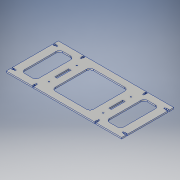
# Autodesk Inventor part: Hopper Bottom Brace
Saved by Autodesk Inventor 2018 (Build 220112000, 112)
## iProperties
Created: 2013-10-08
Part Number: Hopper Bottom Brace
Material: Aluminum 6061
Document SubType Name: Modeling
Designer: Gabriel Smolnycki
Mass: 299.366 g
Surface Area: 651.04 cm^2
Volume: 110.876 cm^3
Density: 2.7 g/cm^3
Appearance: Aluminum - Flat
Sending System: SolidWorks 2017
Last Author: Gabriel Smolnycki
Last Saved: 2017-09-14
Author: Gabriel Smolnycki
Autodesk Inventor part; units mm, degrees
ref_plane "YZ Plane" through (0, 0, 0) normal (1, 0, 0) x (0, 1, 0)
ref_plane "XY Plane" through (0, 0, 0) normal (0, 0, 1) x (1, 0, 0)
ref_plane "Work Plane1" through (0, -4, 0) normal (0, 1, 0) x (-1, 0, 0)
sketch "Sketch1" plane through (0, -4, 0) normal (0, 1, 0) x (-1, 0, 0)
  line L0 (-91.75, 75) -> (-91.75, 72)
  line L1 (88.25, 63) -> (91.75, 63)
  line L2 (163, 57.25) -> (163, 58.25)
  line L3 (91.75, -72) -> (92.75, -72)
  line L4 (-91.75, -63) -> (-91.75, -68)
  line L5 (-163, -58.25) -> (-166, -58.25)
  line L6 (143, -55) -> (143, 55)
  line L7 (-163, 61.75) -> (-166, 61.75)
  line L8 (87.25, 72) -> (87.25, 68)
  line L9 (154, 58.25) -> (159, 58.25)
  line L10 (166, -75) -> (166, -61.75)
  line L11 (-87.25, -68) -> (-88.25, -68)
  line L12 (-159, -58.25) -> (-159, -57.25)
  line L13 (81.5, -20) -> (81.5, 20)
  line L14 (-74.5, 20) -> (-81.5, 20)
  line L15 (-159, 61.75) -> (-159, 62.75)
  line L16 (88.25, 75) -> (-88.25, 75)
  line L17 (159, 62.75) -> (159, 61.75)
  line L18 (159, -62.75) -> (163, -62.75)
  line L19 (-88.25, -75) -> (-88.25, -72)
  line L20 (-159, -61.75) -> (-154, -61.75)
  line L21 (55, -55) -> (55, 55)
  line L22 (-159, 58.25) -> (-154, 58.25)
  line L23 (-87.25, 68) -> (-87.25, 72)
  line L24 (166, 61.75) -> (163, 61.75)
  line L25 (154, -58.25) -> (154, -61.75)
  line L26 (87.25, -72) -> (88.25, -72)
  line L27 (-163, -61.75) -> (-163, -62.75)
  line L28 (-163, 58.25) -> (-163, 57.25)
  line L29 (-91.75, 63) -> (-88.25, 63)
  line L30 (91.75, 72) -> (91.75, 75)
  line L31 (163, -57.25) -> (159, -57.25)
  line L32 (88.25, -63) -> (88.25, -68)
  line L33 (-166, -75) -> (-91.75, -75)
  line L34 (55, 55) -> (-55, 55)
  line L35 (-92.75, 72) -> (-92.75, 68)
  line L36 (91.75, 68) -> (92.75, 68)
  line L37 (166, -58.25) -> (166, 58.25)
  line L38 (92.75, -68) -> (91.75, -68)
  line L39 (-92.75, -68) -> (-92.75, -72)
  line L40 (-101, -55) -> (-101, 55)
  line L41 (101, 55) -> (101, -55)
  line L42 (-91.75, 75) -> (-166, 75)
  line L43 (88.25, 68) -> (88.25, 63)
  line L44 (159, 57.25) -> (163, 57.25)
  line L45 (91.75, -75) -> (91.75, -72)
  line L46 (-88.25, -63) -> (-91.75, -63)
  line L47 (-163, -57.25) -> (-163, -58.25)
  line L48 (74.5, 20) -> (74.5, -20)
  line L49 (101, -55) -> (143, -55)
  line L50 (-163, 62.75) -> (-163, 61.75)
  line L51 (88.25, 72) -> (87.25, 72)
  line L52 (154, 61.75) -> (154, 58.25)
  line L53 (163, -61.75) -> (166, -61.75)
  line L54 (-87.25, -72) -> (-87.25, -68)
  line L55 (-154, -58.25) -> (-159, -58.25)
  line L56 (74.5, -20) -> (81.5, -20)
  line L57 (-154, 61.75) -> (-159, 61.75)
  line L58 (-88.25, 72) -> (-88.25, 75)
  line L59 (163, 62.75) -> (159, 62.75)
  line L60 (159, -61.75) -> (159, -62.75)
  line L61 (-88.25, -75) -> (88.25, -75)
  line L62 (-159, -62.75) -> (-159, -61.75)
  line L63 (-74.5, -20) -> (-74.5, 20)
  line L64 (-159, 57.25) -> (-159, 58.25)
  line L65 (-88.25, 68) -> (-87.25, 68)
  line L66 (166, 61.75) -> (166, 75)
  line L67 (159, -58.25) -> (154, -58.25)
  line L68 (87.25, -68) -> (87.25, -72)
  line L69 (-166, -61.75) -> (-163, -61.75)
  line L70 (-55, -55) -> (55, -55)
  line L71 (-143, 55) -> (-143, -55)
  line L72 (-166, 58.25) -> (-163, 58.25)
  line L73 (-91.75, 68) -> (-91.75, 63)
  line L74 (92.75, 72) -> (91.75, 72)
  line L75 (163, -58.25) -> (163, -57.25)
  line L76 (91.75, -63) -> (88.25, -63)
  line L77 (-91.75, -72) -> (-91.75, -75)
  line L78 (-143, -55) -> (-101, -55)
  line L79 (143, 55) -> (101, 55)
  line L80 (-91.75, 72) -> (-92.75, 72)
  line L81 (91.75, 63) -> (91.75, 68)
  line L82 (163, 58.25) -> (166, 58.25)
  line L83 (92.75, -72) -> (92.75, -68)
  line L84 (-91.75, -68) -> (-92.75, -68)
  line L85 (-166, 75) -> (-166, 61.75)
  line L86 (87.25, 68) -> (88.25, 68)
  line L87 (159, 58.25) -> (159, 57.25)
  line L88 (91.75, -75) -> (166, -75)
  line L89 (-88.25, -68) -> (-88.25, -63)
  line L90 (-159, -57.25) -> (-163, -57.25)
  line L91 (81.5, 20) -> (74.5, 20)
  line L92 (-159, 62.75) -> (-163, 62.75)
  line L93 (88.25, 75) -> (88.25, 72)
  line L94 (159, 61.75) -> (154, 61.75)
  line L95 (163, -62.75) -> (163, -61.75)
  line L96 (-88.25, -72) -> (-87.25, -72)
  line L97 (-154, -61.75) -> (-154, -58.25)
  line L98 (-81.5, 20) -> (-81.5, -20)
  line L99 (-81.5, -20) -> (-74.5, -20)
  line L100 (-154, 58.25) -> (-154, 61.75)
  line L101 (-87.25, 72) -> (-88.25, 72)
  line L102 (163, 61.75) -> (163, 62.75)
  line L103 (154, -61.75) -> (159, -61.75)
  line L104 (88.25, -72) -> (88.25, -75)
  line L105 (-163, -62.75) -> (-159, -62.75)
  line L106 (-163, 57.25) -> (-159, 57.25)
  line L107 (-88.25, 63) -> (-88.25, 68)
  line L108 (166, 75) -> (91.75, 75)
  line L109 (159, -57.25) -> (159, -58.25)
  line L110 (88.25, -68) -> (87.25, -68)
  line L111 (-166, -61.75) -> (-166, -75)
  line L112 (-55, 55) -> (-55, -55)
  line L113 (-92.75, 68) -> (-91.75, 68)
  line L114 (92.75, 68) -> (92.75, 72)
  line L115 (166, -58.25) -> (163, -58.25)
  line L116 (91.75, -68) -> (91.75, -63)
  line L117 (-92.75, -72) -> (-91.75, -72)
  line L118 (-166, 58.25) -> (-166, -58.25)
  line L119 (-101, 55) -> (-143, 55)
  constraints: 240 end point, 84 equal length, 60 horizontal, 60 vertical, 14 collinear
extrude "Extrusion1" add sketch "Sketch1" along normal blind 4.064
fillet "Fillet1" radius 10 12 edges at (101, -1.968, 55) (-55, -1.968, -55) (-143, -1.968, -55) (101, -1.968, -55) (-55, -1.968, 55) (-143, -1.968, 55) (143, -1.968, -55) (55, -1.968, -55) (-101, -1.968, -55) (143, -1.968, 55) (55, -1.968, 55) (-101, -1.968, 55)
hole "Hole4" at (78, -4, 40) direction (0, 1, 0) diameter 3.5 depth 4.064
hole "Hole3" at (78, -4, -40) direction (0, 1, 0) diameter 3.5 depth 4.064
sketch "Sketch3" plane through (0, -4, 0) normal (0, 1, 0) x (-1, 0, 0)
  point P0 (-78, -40)
hole "Hole2" at (-78, -4, 40) direction (0, 1, 0) diameter 3.5 depth 4.064
sketch "Sketch2" plane through (0, -4, 0) normal (0, 1, 0) x (-1, 0, 0)
  point P0 (-78, 40)
hole "Hole1" at (-78, -4, -40) direction (0, 1, 0) diameter 3.5 depth 4.064
sketch "Sketch4" plane through (0, -4, 0) normal (0, 1, 0) x (-1, 0, 0)
  point P0 (78, 40)
sketch "Sketch5" plane through (0, -4, 0) normal (0, 1, 0) x (-1, 0, 0)
  point P0 (78, -40)
body "Solid3"
